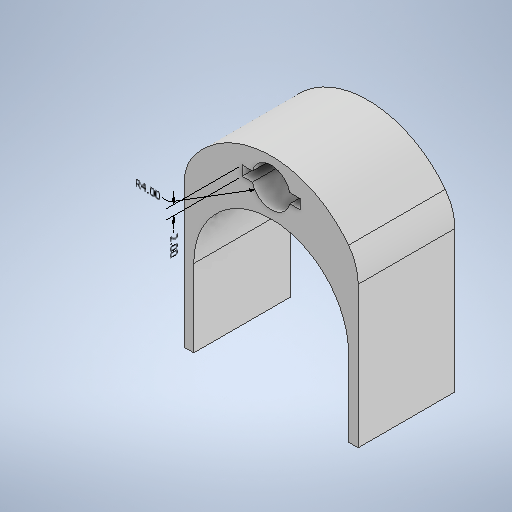
# Autodesk Inventor part: شوكه حيه
Saved by Autodesk Inventor 2025.4 (Build 294407000, 407)
## iProperties
Created: 2026-04-06
Part Number: شوكه حيه
Material: Generic
Document SubType Name: Modeling
Designer: Amir
Density: 1 g/cm^3
Appearance: Default
Author: Amir
## iProperties of the stored document final sorrting_3DPrint.ipt
Created: 2026-04-09
Part Number: final sorrting_3DPrint
Material: Generic
Document SubType Name: Modeling
Designer: Amir
Density: 1 g/cm^3
Appearance: Default
Author: Amir
Autodesk Inventor part; units mm, degrees
ref_plane "YZ Plane" through (0, 0, 0) normal (1, 0, 0) x (0, 1, 0)
ref_plane "XZ Plane" through (0, 0, 0) normal (0, 1, 0) x (-1, 0, 0)
ref_plane "XY Plane" through (0, 0, 0) normal (0, 0, 1) x (1, 0, 0)
sketch "Sketch1" plane through (0, 0, 0) normal (0, 0, 1) x (1, 0, 0)
  arc A0 (16, 0) -> (-16, 0) centre (0, 0) ccw
  line L0 (-16, 0) -> (-16, -16)
  line L1 (16, 0) -> (16, -16)
  line L2 (-16, -16) -> (-18, -16)
  line L3 (-18, -16) -> (-18, 16)
  line L4 (16, -16) -> (18, -16)
  line L5 (18, -16) -> (18, 16)
  circle A1 centre (0, 21.6411) radius 4
  arc A2 (18, 16) -> (-18, 16) centre (0, 7.2822) ccw
  line L6 (-6, 20.6411) -> (6, 20.6411)
  line L7 (6, 20.6411) -> (6, 22.6411)
  line L8 (6, 22.6411) -> (-6, 22.6411)
  line L9 (-6, 22.6411) -> (-6, 20.6411)
  line L10 (-6, 20.6411) -> (6, 22.6411) construction
  line L11 (6, 20.6411) -> (-6, 22.6411) construction
  point P0 (3.873, 20.6411)
  point P1 (-3.873, 20.6411)
  point P2 (-3.873, 22.6411)
  point P3 (3.873, 22.6411)
  dimension "d6" = 32
  dimension "d7" = 2
  dimension "d8" = 2
  dimension "d10" = 8
  dimension "d11" = 12
  dimension "d12" = 2
  dimension "d13" = 20
  constraints: 24 end point, 4 point on circle, 3 centre point, 3 horizontal, 3 parallel, 3 perpendicular, 2 midpoint, 2 tangent, 1 vertical
  measures "d6" diameter of A0
  measures "d7" distance of L0.end L2.end
  measures "d8" distance of L1.end L4.end
  measures "d10" diameter of A1
  measures "d11" distance of L8.end L7.end
  measures "d12" distance of L7.end L6.end
  measures "d13" radius of A2
extrude "Extrusion1" add sketch "Sketch1" along normal blind 20
fillet "Fillet1" radius 10 2 edges at (18, 16, 10) (-18, 16, 10)
body "Solid1"
